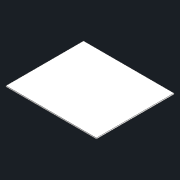
# Autodesk Inventor part: s_carbon_plate1
Saved by Autodesk Inventor 2021 (Build 250183000, 183)
## iProperties
Created: 2021-08-20
Part Number: s_carbon_plate1
Material: ABS プラスチック
Document SubType Name: Sheet Metal
Designer: yuta0
Density: 1.06 g/cm^3
Sheet Metal Rule: Default_mm
Appearance: 滑らか - 白
Author: yuta0
Autodesk Inventor part; units mm, degrees
ref_plane "YZ Plane" through (0, 0, 0) normal (1, 0, 0) x (0, 1, 0)
ref_plane "XZ Plane" through (0, 0, 0) normal (0, 1, 0) x (-1, 0, 0)
ref_plane "XY Plane" through (0, 0, 0) normal (0, 0, 1) x (1, 0, 0)
sketch "スケッチ1" plane through (0, 0, 0) normal (0, 1, 0) x (-1, 0, 0)
  line L0 (-87.5, 75) -> (87.5, 75)
  line L1 (87.5, 75) -> (87.5, -75)
  line L2 (87.5, -75) -> (-87.5, -75)
  line L3 (-87.5, -75) -> (-87.5, 75)
  line L4 (-87.5, 75) -> (87.5, -75) construction
  line L5 (87.5, 75) -> (-87.5, -75) construction
  point P0 (0, 0)
  dimension "d0" = 150
  dimension "d1" = 175
  measures "d0" distance of L0.end L1.end
  measures "d1" distance of L0.start L0.end
extrude "プレート1" add sketch "スケッチ1" along normal blind 2
equation "\"d2\" = Thickness"
equation "\"BendRadius\" = Thickness"
equation "\"BendReliefWidth\" = Thickness"
equation "\"BendReliefDepth\" = 0.5 * Thickness"
equation "\"CornerReliefSize\" = 4 * Thickness"
equation "\"MinimumRemnant\" = 2 * Thickness"
equation "\"TransitionRadius\" = BendRadius"
equation "\"JacobiRadiusSize\" = BendRadius"
equation "\"GapSize\" = Thickness"
equation "\"Thickness\" = 2"
